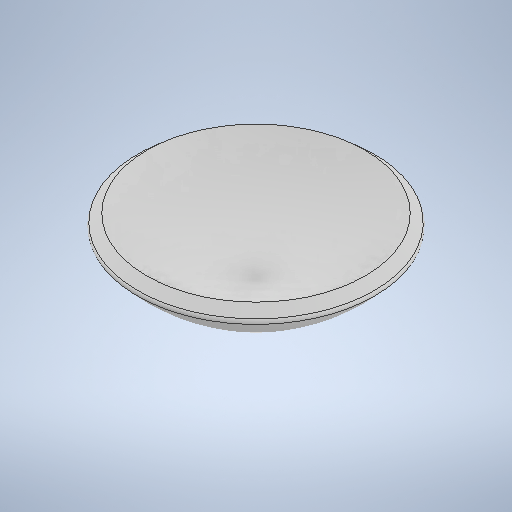
# Autodesk Inventor part: Front Shield TPS
Saved by Autodesk Inventor 2026.2 (Build 302298000, 298)
## iProperties
Created: 2026-01-18
Part Number: Front Shield TPS
Material: Generic
Document SubType Name: Modeling
Designer: daryu
Density: 1 g/cm^3
Appearance: Default
Author: daryu
Autodesk Inventor part; units mm, degrees
ref_plane "YZ Plane" through (0, 0, 0) normal (1, 0, 0) x (0, 1, 0)
ref_plane "XZ Plane" through (0, 0, 0) normal (0, 1, 0) x (-1, 0, 0)
ref_plane "XY Plane" through (0, 0, 0) normal (0, 0, 1) x (1, 0, 0)
sketch "Sketch2" plane through (0, 0, 0) normal (0, 0, 1) x (1, 0, 0)
  arc A0 (0, 0) -> (37.0674, 19.7262) centre (-4.6377, 53.4043) ccw
  line L0 (0, 0) -> (0, 10)
  arc A1 (0, 5) -> (33.5015, 22.8194) centre (-10.6686, 65.4597) ccw
  line L1 (37.0674, 19.7262) -> (33.5015, 22.8194)
  point P0 (35.2844, 21.2728)
  dimension "d10" = 10
  dimension "d12" = 61.3938
  dimension "d13" = 53.6053
  dimension "d14" = 4.7205
  dimension "d15" = 19.7262
  dimension "d16" = 22.8194
  dimension "d17" = 35.2844
  constraints: 4 end point, 4 point on circle, 2 centre point, 2 midpoint, 1 vertical
  measures "d10" distance of L0.start L0.end
  measures "d12" radius of A1
  measures "d13" radius of A0
  measures "d14" distance of L1.start L1.end
  measures "d15" vertical distance of L0.start L1.start
  measures "d16" vertical distance of L0.start L1.end
  measures "d17" horizontal distance of L0.start point (35.284, 21.273)
revolve "Revolution1" add sketch "Sketch2" angle 360 about axis through (0, 0, 0) along (0, 1, 0)
fillet "Fillet1" radius 1 1 edges at (-37.0674, 19.7262, 0)
body "Solid1"
